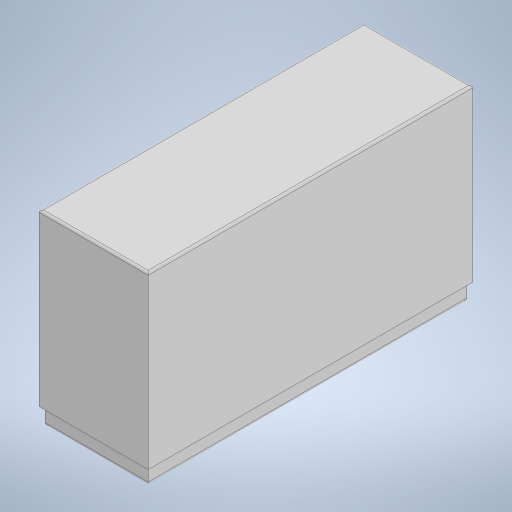
# Autodesk Inventor part: Caja bateria
Saved by Autodesk Inventor 2024.2 (Build 282272000, 272)
## iProperties
Created: 2024-11-30
Part Number: Caja bateria
Material: Genérico
Document SubType Name: Modeling
Designer: sergi
Density: 1 g/cm^3
Appearance: Valor por defecto
Author: sergi
Autodesk Inventor part; units mm, degrees
ref_plane "YZ Plane" through (0, 0, 0) normal (1, 0, 0) x (0, 1, 0)
ref_plane "XZ Plane" through (0, 0, 0) normal (0, 1, 0) x (-1, 0, 0)
ref_plane "XY Plane" through (0, 0, 0) normal (0, 0, 1) x (1, 0, 0)
sketch "Boceto1" plane through (0, 0, 0) normal (0, 1, 0) x (-1, 0, 0)
  line L0 (-25.25, 75.25) -> (25.25, 75.25)
  line L1 (25.25, 75.25) -> (25.25, -75.25)
  line L2 (25.25, -75.25) -> (-25.25, -75.25)
  line L3 (-25.25, -75.25) -> (-25.25, 75.25)
  line L4 (-25.25, 75.25) -> (25.25, -75.25) construction
  line L5 (25.25, 75.25) -> (-25.25, -75.25) construction
  line L6 (22.25, -72.25) -> (22.25, 72.25)
  line L7 (22.25, 72.25) -> (-22.25, 72.25)
  line L8 (-22.25, 72.25) -> (-22.25, -72.25)
  line L9 (-22.25, -72.25) -> (22.25, -72.25)
  point P0 (0, 0)
  dimension "d0" = 50.5
  dimension "d1" = 150.5
  dimension "d2" = 3
  dimension "d3" = 44.5
  constraints: 20 end point, 4 parallel, 2 midpoint, 2 perpendicular, 1 horizontal, 3 other
  measures "d0" distance of L1.end L2.end
  measures "d1" distance of L0.end L1.end
  measures "d2" distance between parallel lines of L1 L6
  measures "d3" distance between parallel lines of L8 L6
extrude "Extrusión1" add sketch "Boceto1" along normal blind 79
sketch "Boceto2" plane through (0, 79, 0) normal (0, 1, 0) x (1, 0, 0)
  line L0 (-22.25, -72.25) -> (-22.25, 72.25) projected
  line L1 (25.25, 75.25) -> (-25.25, 75.25) projected
  line L2 (-25.25, 75.25) -> (-25.25, -75.25) projected
  line L3 (-25.25, -75.25) -> (25.25, -75.25) projected
  line L4 (25.25, -75.25) -> (25.25, 75.25) projected
  line L5 (-22.25, 72.25) -> (22.25, 72.25) projected
  line L6 (22.25, 72.25) -> (22.25, -72.25) projected
  line L7 (22.25, -72.25) -> (-22.25, -72.25) projected
  line L8 (-22.25, -72.25) -> (-22.25, 72.25) projected
  point P0 (0, 0)
  point P1 (-22.25, 72.25)
extrude "Extrusión2" add sketch "Boceto2" against normal blind 3 contours L0 L5 L6 L7
fillet "Empalme1" radius 1 4 edges at (0, 79, 75.25) (25.25, 79, 0) (-25.25, 79, 0) (0, 79, -75.25)
sketch "Boceto3" plane through (0, 0, 0) normal (0, -1, 0) x (1, 0, 0)
  line L0 (25.25, -75.25) -> (-25.25, -75.25) projected
  line L1 (25.25, 75.25) -> (25.25, -75.25) projected
  line L2 (-25.25, 75.25) -> (25.25, 75.25) projected
  line L3 (-25.25, -75.25) -> (-25.25, 75.25) projected
  line L4 (-22.25, -72.25) -> (22.25, -72.25) projected
  line L5 (-22.25, 72.25) -> (-22.25, -72.25) projected
  line L6 (22.25, 72.25) -> (-22.25, 72.25) projected
  line L7 (22.25, -72.25) -> (22.25, 72.25) projected
  line L8 (23.85, 73.85) -> (-23.85, 73.85)
  line L9 (-23.85, 73.85) -> (-23.85, -73.85)
  line L10 (-23.85, -73.85) -> (23.85, -73.85)
  line L11 (23.85, -73.85) -> (23.85, 73.85)
  point P0 (0, 0)
  dimension "d9" = 1.6
  constraints: 8 end point, 3 other
  measures "d9" distance between parallel lines of L7 L11
extrude "Extrusión3" add sketch "Boceto3" along normal blind 8 contours L11 L10 L9 L8
fillet "Empalme2" radius 1.6 4 edges at (-23.85, -8, 0) (0, -8, 73.85) (23.85, -8, 0) (0, -8, -73.85)
fillet "Empalme3" radius 1.6 4 edges at (22.25, 76, 0) (0, 76, 72.25) (0, 76, -72.25) (-22.25, 76, 0)
